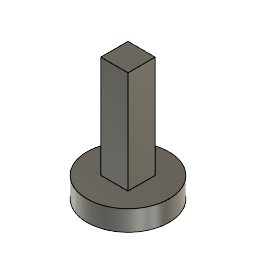
robotic pick and place (Assembly) (Autodesk Fusion 360 archive; units mm, degrees)
design "robotic pick and place"
part number: 2026-03-22-09-44-44-743
Autodesk Fusion 360 part; units mm, degrees
sketch "Sketch1" plane through (0, 0, 0) normal (0, 0, 1) x (1, 0, 0)
  circle A0 centre (0, 0) radius 60
  dimension "d1" = 120
  constraint coincident A0.centre origin
  measures "d1" diameter of A0
extrude "Extrude1" add sketch "Sketch1" along normal blind 30
sketch "Sketch2" plane through (0, 0, 30) normal (0, 0, 1) x (-1, 0, 0)
  circle A0 centre (0, 0) radius 60
  line L0 (20, 20) -> (-20, 20)
  line L1 (-20, 20) -> (-20, -20)
  line L2 (-20, -20) -> (20, -20)
  line L3 (20, -20) -> (20, 20)
  line L4 (20, 20) -> (-20, -20) construction
  line L5 (-20, 20) -> (20, -20) construction
  dimension "d4" = 40
  dimension "d5" = 40
  constraint horizontal L0
  constraint perpendicular L0 L1
  constraint parallel L0 L2
  constraint parallel L1 L3
  constraint coincident L4 A0.centre
  constraint coincident L5 A0.centre
  constraint coincident A0.centre origin
  measures "d4" distance of L1.end L2.end
  measures "d5" distance of L0.end L1.end
extrude "Extrude2" add sketch "Sketch2" along normal blind 150 contours L0 L1 L2 L3
sketch "Sketch3" plane through (0, 0, 0) normal (0, 1, 0) x (1, 0, 0)
sketch "Sketch4" plane through (0, 0, 0) normal (0, 1, 0) x (1, 0, 0)

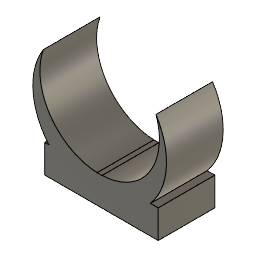
design "Gripper"
part number: 2026-03-22-16-25-26-350
Autodesk Fusion 360 part; units mm, degrees
sketch "Sketch1" plane through (0, 0, 0) normal (0, 0, 1) x (1, 0, 0)
  line L0 (142.856, -0.1333) -> (102.856, -0.1333)
  line L1 (102.856, -0.1333) -> (102.856, 19.8667)
  line L2 (102.856, 19.8667) -> (142.856, 19.8667)
  line L3 (142.856, 19.8667) -> (142.856, -0.1333)
  dimension "d1" = 40
  dimension "d2" = 20
  constraint horizontal L0
  constraint vertical L1
  constraint horizontal L2
  constraint vertical L3
  measures "d1" distance of L0.start L0.end
  measures "d2" distance of L0.start L2.end
extrude "Extrude1" add sketch "Sketch1" along normal blind 10
sketch "Sketch2" plane through (0, -0.1333, 0) normal (0, -1, 0) x (1, 0, 0)
  line L0 (102.856, 0) -> (142.856, 0)
  line L1 (142.856, 0) -> (142.856, 10)
  line L2 (142.856, 10) -> (102.856, 10)
  line L3 (102.856, 10) -> (102.856, 0)
  arc A0 (102.443, 38.096) -> (142.0192, 38.096) centre (122.2311, 31.0031) ccw
  arc A1 (102.443, 38.096) -> (142.0192, 38.096) centre (122.2311, 25.3257) ccw
sketch "Sketch3" plane through (0, -0.1333, 0) normal (0, -1, 0) x (1, 0, 0)
extrude "Extrude2" add sketch "Sketch2" against normal blind 20 contours L2 A0 A1 | L2 A0 A1 picked at (104.808, 12.829) picked at (139.6542, 12.829)

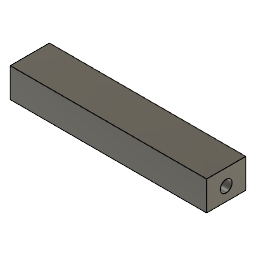
design "link1"
part number: 2026-03-22-09-57-37-753
Autodesk Fusion 360 part; units mm, degrees
sketch "Sketch1" plane through (0, 0, 0) normal (0, 1, 0) x (1, 0, 0)
  line L0 (0, 0) -> (200, 0)
  line L1 (200, 0) -> (200, -30)
  line L2 (200, -30) -> (0, -30)
  line L3 (0, -30) -> (0, 0)
  dimension "d1" = 200
  dimension "d2" = 30
  constraint horizontal L0
  constraint vertical L1
  constraint horizontal L2
  constraint vertical L3
  constraint coincident L0.start L3.end
  measures "d1" distance of L0.start L0.end
  measures "d2" distance of L0.start L2.end
extrude "Extrude1" add sketch "Sketch1" along normal mid plane 40
sketch "Sketch2" plane through (200, 0, 0) normal (1, 0, 0) x (0, 1, 0)
  line L0 (-20, 0) -> (20, 0)
  line L1 (20, 0) -> (20, 30)
  line L2 (20, 30) -> (-20, 30)
  line L3 (-20, 30) -> (-20, 0)
  circle A0 centre (0, 13.7868) radius 6
  dimension "d5" = 12
  measures "d5" diameter of A0
extrude "Extrude2" cut sketch "Sketch2" against normal blind 200 contours A0
move_body "Move1" bodies 1 to x (1, 0, 0) y (0, 1, 0) z (0, 0, 1) at (100, 0, 0)
sketch "Sketch3" plane through (0, 0, 0) normal (0, 1, 0) x (1, 0, 0)

design "link2"
part number: 2026-03-22-10-04-24-623
Autodesk Fusion 360 part; units mm, degrees
sketch "Sketch1" plane through (0, 0, 0) normal (0, 1, 0) x (1, 0, 0)
  line L0 (0, 0) -> (150, 0)
  line L1 (150, 0) -> (150, -25)
  line L2 (150, -25) -> (0, -25)
  line L3 (0, -25) -> (0, 0)
  dimension "d1" = 150
  dimension "d2" = 25
  constraint horizontal L0
  constraint vertical L1
  constraint horizontal L2
  constraint vertical L3
  constraint coincident L0.start L3.end
  measures "d1" distance of L0.start L0.end
  measures "d2" distance of L0.start L2.end
extrude "Extrude1" add sketch "Sketch1" along normal mid plane 40
sketch "Sketch2" plane through (0, -20, 0) normal (0, -1, 0) x (1, 0, 0)
  line L0 (150, 25) -> (0, 25)
  line L1 (0, 25) -> (0, 0)
  line L2 (0, 0) -> (150, 0)
  line L3 (150, 0) -> (150, 25)
sketch "Sketch3" plane through (0, -20, 0) normal (0, -1, 0) x (1, 0, 0)
sketch "Sketch4" plane through (0, -20, 0) normal (0, -1, 0) x (1, 0, 0)
sketch "Sketch5" plane through (0, 0, 0) normal (-1, 0, 0) x (0, -1, 0)
  line L0 (20, 25) -> (-20, 25)
  line L1 (-20, 25) -> (-20, 0)
  line L2 (-20, 0) -> (20, 0)
  line L3 (20, 0) -> (20, 25)
  circle A0 centre (0, 13) radius 5
  dimension "d5" = 10
  measures "d5" diameter of A0
extrude "Extrude2" cut sketch "Sketch5" against normal blind 150 keep common part
